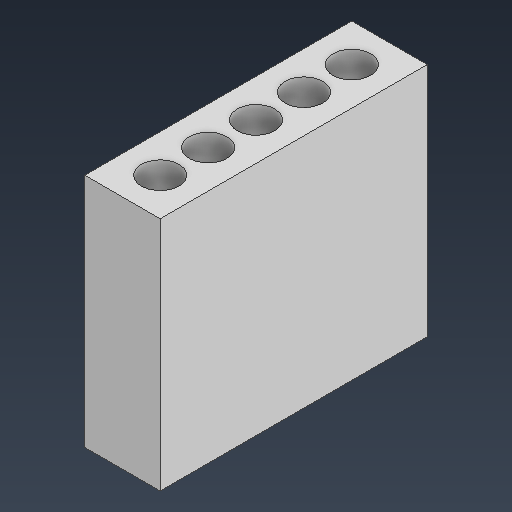
# Autodesk Inventor part: Encoder Header Spacer 2
Saved by Autodesk Inventor 2025.3 (Build 293356000, 356)
## iProperties
Created: 2025-09-25
Part Number: Encoder Header Spacer 2
Material: Generic
Document SubType Name: Modeling
Designer: tolga
Density: 1 g/cm^3
Appearance: Default
Author: tolga
Autodesk Inventor part; units mm, degrees
ref_plane "YZ Plane" through (0, 0, 0) normal (1, 0, 0) x (0, 1, 0)
ref_plane "XZ Plane" through (0, 0, 0) normal (0, 1, 0) x (-1, 0, 0)
ref_plane "XY Plane" through (0, 0, 0) normal (0, 0, 1) x (1, 0, 0)
sketch "Sketch1" plane through (0, 0, 0) normal (0, 1, 0) x (-1, 0, 0)
  circle A0 centre (0, 0) radius 1
  line L0 (2, 2) -> (-2, 2)
  line L1 (-2, 2) -> (-2, -12.16)
  line L2 (-2, -12.16) -> (2, -12.16)
  line L3 (2, -12.16) -> (2, 2)
  circle A1 centre (0, -2.54) radius 1
  circle A2 centre (0, -5.08) radius 1
  circle A3 centre (0, -7.62) radius 1
  circle A4 centre (0, -10.16) radius 1
  dimension "d0" = 2
  dimension "d3" = 2.54
  dimension "d8" = 1
  dimension "d9" = 1
  dimension "d10" = 1
  dimension "d11" = 1
  constraints: 8 end point, 5 centre point, 2 parallel, 1 coincident, 1 horizontal, 1 perpendicular, 1 vertical, 8 other
  measures "d0" diameter of A0
  measures "d3" distance of A0.centre A1.centre
  measures "d8" distance edge to line of A0 L3
  measures "d9" distance edge to line of A0 L0
  measures "d10" distance edge to line of A0 L1
  measures "d11" distance edge to line of A4 L2
extrude "Extrusion1" add sketch "Sketch1" along normal blind 12.5
equation "\"d9\" = d8"
equation "\"d10\" = d8"
equation "\"d11\" = d8"
body "Solid1"
